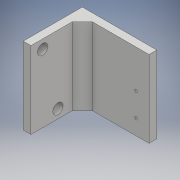
# Autodesk Inventor part: Estrutura - SensorX
Saved by Autodesk Inventor 2017 (Build 210142000, 142)
## iProperties
Created: 2020-09-29
Part Number: Estrutura - SensorX
Material: Generic
Document SubType Name: Modeling
Designer: ale
Density: 1 g/cm^3
Appearance: Default
Author: ale
Autodesk Inventor part; units mm, degrees
ref_plane "YZ Plane" through (0, 0, 0) normal (1, 0, 0) x (0, 1, 0)
ref_plane "XZ Plane" through (0, 0, 0) normal (0, 1, 0) x (-1, 0, 0)
ref_plane "XY Plane" through (0, 0, 0) normal (0, 0, 1) x (1, 0, 0)
sketch "Sketch1" plane through (0, 0, 0) normal (0, 0, 1) x (1, 0, 0)
  line L0 (0, -4) -> (0, -20)
  line L1 (4, 0) -> (26, 0)
  line L2 (26, 3) -> (-3, 3)
  line L3 (-3, 3) -> (-3, -20)
  line L4 (26, 3) -> (26, 0)
  line L5 (0, -20) -> (-3, -20)
  line L6 (4, 0) -> (0, -4)
  point P0 (0, 0)
  point P1 (0, 0)
  dimension "d0" = 20
  dimension "d1" = 26
  dimension "d2" = 3
  dimension "d5" = 4
  dimension "d6" = 4
  constraints: 14 end point, 4 point on line, 2 vertical, 1 horizontal, 1 perpendicular, 1 other
  measures "d0" distance of point (0, 0) L0.end
  measures "d1" distance of point (0, 0) L1.end
  measures "d2" distance between parallel lines of L1 L2
  measures "d5" distance of L1.start point (0, 0)
  measures "d6" distance of L0.start point (0, 0)
extrude "Extrusion1" add sketch "Sketch1" along normal blind 30
sketch "Sketch2" plane through (-3, 3, 0) normal (0, 1, 0) x (1, 0, 0)
  line L0 (29, 0) -> (0, 0) projected
  line L1 (29, 0) -> (29, -30) projected
  point P0 (3, 0)
  point P1 (24, -6)
  point P2 (24, -15.2)
  dimension "d9" = 9.2
  dimension "d10" = 6
  dimension "d11" = 5
  dimension "d12" = 5
  measures "d9" distance of point (24, -15.2) point (24, -6)
  measures "d10" distance from line of point (24, -6) L0
  measures "d11" distance from line of point (24, -6) L1
  measures "d12" distance from line of L1 point (24, -15.2)
hole "Hole1" at (21, 3, 6) at (21, 3, 15.2) direction (0, -1, 0) diameter 1 end through all
sketch "Sketch3" plane through (0, -20, 0) normal (1, 0, 0) x (0, 0, -1)
  line L0 (0, 0) -> (0, 16) projected
  line L1 (0, 0) -> (-30, 0) projected
  line L2 (0, 16) -> (-30, 16) projected
  point P0 (0, 20)
  point P1 (-3.5, 10.5)
  point P2 (-26.5, 4.5)
  dimension "d20" = 3.5
  dimension "d29" = 5.5
  dimension "d30" = 23
  dimension "d31" = 6
  measures "d20" distance from line of L0 point (-3.5, 10.5)
  measures "d29" distance from line of L2 point (-3.5, 10.5)
  measures "d30" horizontal distance of point (-26.5, 4.5) point (-3.5, 10.5)
  measures "d31" vertical distance of point (-26.5, 4.5) point (-3.5, 10.5)
hole "Hole2" at (0, -9.5, 3.5) at (0, -15.5, 26.5) direction (-1, 0, 0) diameter 4 end through all
equation "\"d6\" = d5"
body "Solid1"
